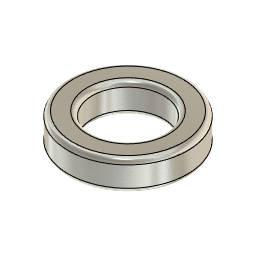
MG996R_Bushing_Teflon v4 (Autodesk Fusion 360 design; units mm, degrees)
Autodesk Fusion 360 part; units mm, degrees
sketch "Sketch1" plane through (0, 0, 0) normal (0, 0, 1) x (1, 0, 0)
  circle A0 centre (0, 0) radius 3
  circle A1 centre (0, 0) radius 5
  dimension "d1" = 10
  dimension "d2" = 6
  constraint coincident A0.centre A1.centre
  constraint concentric A0 A1
  measures "d1" diameter of A1
  measures "d2" diameter of A0
extrude "Extrude1" add sketch "Sketch1" along normal blind 2.5
fillet "Fillet1" radius 0.4 4 edges at (-2.797, 1.0848, 2.5) (-2.797, 1.0848, 0) (-4.6616, -1.8081, 2.5) (-4.6616, -1.8081, 0)
